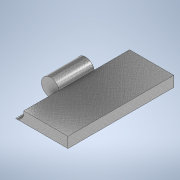
# Autodesk Inventor part: Clip1
Saved by Autodesk Inventor 2021 (Build 250183000, 183)
## iProperties
Created: 2023-04-06
Part Number: Clip1
Material: Stainless Steel
Document SubType Name: Modeling
Designer: EF0481
Density: 8 g/cm^3
Appearance: Honed
Author: EF0481
Autodesk Inventor part; units mm, degrees
ref_plane "YZ Plane" through (0, 0, 0) normal (1, 0, 0) x (0, 1, 0)
ref_plane "XZ Plane" through (0, 0, 0) normal (0, 1, 0) x (-1, 0, 0)
ref_plane "XY Plane" through (0, 0, 0) normal (0, 0, 1) x (1, 0, 0)
sketch "Sketch1" plane through (0, 0, 0) normal (0, 0, 1) x (1, 0, 0)
  line L0 (0, 0) -> (15, 0)
  line L1 (15, 0) -> (15, 3)
  line L2 (15, 3) -> (0, 3)
  line L3 (0, 3) -> (0, 0)
  circle A0 centre (0, 2.5) radius 2.5
  point P0 (0, 1.5)
  point P1 (2.4495, 3)
  dimension "d0" = 15
  dimension "d1" = 3
  dimension "d2" = 5
  constraints: 8 end point, 2 parallel, 1 centre point, 1 horizontal, 1 midpoint, 1 perpendicular, 1 tangent, 1 vertical alignment
  measures "d0" distance of L2.end L1.end
  measures "d1" distance of L1.end L0.end
  measures "d2" diameter of A0
extrude "Extrusion1" add sketch "Sketch1" against normal blind 30
sketch "Sketch2" plane through (0, 0, 0) normal (0, 0, 1) x (1, 0, 0)
  arc A0 (2.4495, 3) -> (0, 0) centre (0, 2.5) ccw projected
  circle A1 centre (0.0044, 2.5032) radius 2.51
  dimension "d5" = 5.02
  constraints: 2 coincident, 1 centre point
  measures "d5" diameter of A1
extrude "Extrusion2" cut sketch "Sketch2" against normal blind 10
pattern_linear "Rectangular Pattern1" count 2 spacing 20 along (0, 0, -1) of "Extrusion2"
body "Solid1"
